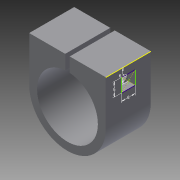
# Autodesk Inventor part: slik_clamp_head38_collar
Saved by Autodesk Inventor 2013 (Build 170138000, 138)
## iProperties
Created: 2013-01-30
Part Number: slik_clamp_head38_collar
Material: Generic
Document SubType Name: Modeling
Designer: Mahisorn
Density: 1 g/cm^3
Author: Mahisorn
Autodesk Inventor part; units mm, degrees
ref_plane "YZ Plane" through (0, 0, 0) normal (1, 0, 0) x (0, 1, 0)
ref_plane "XZ Plane" through (0, 0, 0) normal (0, 1, 0) x (-1, 0, 0)
ref_plane "XY Plane" through (0, 0, 0) normal (0, 0, 1) x (1, 0, 0)
sketch "Sketch1" plane through (0, 0, 0) normal (0, 1, 0) x (-1, 0, 0)
  arc A0 (-1, 13.4629) -> (1, 13.4629) centre (0, 0) ccw
  arc A1 (-17, 0) -> (17, 0) centre (0, 0) ccw
  line L0 (17, 0) -> (17, 19.8)
  line L1 (-17, 19.8) -> (-17, 0)
  line L2 (-1, 19.8) -> (-1, 13.4629)
  line L3 (1, 19.8) -> (1, 13.4629)
  line L4 (17, 19.8) -> (1, 19.8)
  line L5 (-1, 19.8) -> (-17, 19.8)
  dimension "d0" = 27
  dimension "d1" = 34
  constraints: 12 end point, 4 point on circle, 2 centre point, 2 coincident, 2 parallel
  measures "d0" diameter of A0
  measures "d1" diameter of A1
extrude "Extrusion1" add sketch "Sketch1" along normal blind 20
sketch "Sketch2" plane through (17, 0, 19.8) normal (1, 0, 0) x (0, 0, -1)
  line L0 (0, 0) -> (0, 20) projected
  line L1 (3.52, 13) -> (9.52, 13)
  line L2 (9.52, 13) -> (9.52, 7)
  line L3 (9.52, 7) -> (3.52, 7)
  line L4 (3.52, 7) -> (3.52, 13)
  line L5 (3.52, 13) -> (9.52, 7) construction
  line L6 (9.52, 13) -> (3.52, 7) construction
  point P0 (6.52, 10)
  dimension "d7" = 6.52
  dimension "d15" = 6
  dimension "d16" = 6
  constraints: 12 end point, 2 midpoint, 2 parallel, 1 horizontal, 1 perpendicular
  measures "d7" distance from line of L0 point (6.52, 10)
  measures "d15" distance of L2.end L3.end
  measures "d16" distance of L1.end L2.end
hole "Hole1" at (17, 10, 13.28) direction (-1, 0, 0) diameter 5.791 end through all clearance for "Flat Head Machine Screw (82)" size "#12" standard "Ansi Unified Screw Threads"
extrude "Extrusion2" cut sketch "Sketch2" against normal blind 3.3
body "Solid1"
